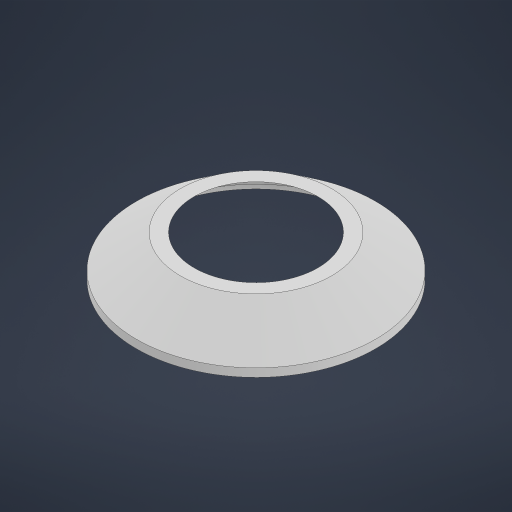
# Autodesk Inventor part: bottom
Saved by Autodesk Inventor 2024 (Build 280153000, 153)
## iProperties
Created: 2024-01-23
Part Number: bottom
Material: Generic
Document SubType Name: Modeling
Designer: madis
Density: 1 g/cm^3
Appearance: Default
Author: madis
Autodesk Inventor part; units mm, degrees
ref_plane "YZ Plane" through (0, 0, 0) normal (1, 0, 0) x (0, 1, 0)
ref_plane "XZ Plane" through (0, 0, 0) normal (0, 1, 0) x (-1, 0, 0)
ref_plane "XY Plane" through (0, 0, 0) normal (0, 0, 1) x (1, 0, 0)
sketch "Sketch1" plane through (0, 0, 0) normal (0, 0, 1) x (1, 0, 0)
  line L0 (29, 2) -> (18.3333, 10)
  line L1 (18.3333, 10) -> (15, 10)
  line L2 (15, 10) -> (27, 1)
  line L3 (29, 2) -> (29, 0)
  line L4 (29, 0) -> (27, 0)
  line L5 (27, 0) -> (27, 1)
  line L6 (0, 0) -> (0, 20.8635) construction
  dimension "d0" = 2
  dimension "d1" = 2
  dimension "d2" = 2
  dimension "d3" = 1
  dimension "d4" = 10
  dimension "d5" = 0
  dimension "d6" = 15
  constraints: 14 end point, 2 parallel, 2 perpendicular, 2 vertical
  measures "d0" distance of L0.start L3.end
  measures "d1" distance of L3.end L4.end
  measures "d2" distance between parallel lines of L2 L0
  measures "d3" distance of L4.end L2.end
  measures "d4" distance between parallel lines of L4 L1
  measures "d5" distance from line of L4 L6.start
  measures "d6" horizontal distance of L6.start L1.end
revolve "Revolution1" add sketch "Sketch1" angle 360 about axis through (0, 0, 0) along (0, 1, 0)
body "Solid1"
